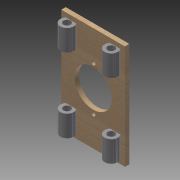
# Autodesk Inventor part: X_Carriage_WithBearings
Saved by Autodesk Inventor 2014 (Build 180170000, 170)
## iProperties
Created: 2013-12-16
Part Number: X_Carriage_WithBearings
Material: Ash
Document SubType Name: Modeling
Designer: Bram
Density: 0.641 g/cm^3
Appearance: Ash Door
Author: Bram
Autodesk Inventor part; units mm, degrees
ref_plane "YZ Plane" through (0, 0, 0) normal (1, 0, 0) x (0, 1, 0)
ref_plane "XZ Plane" through (0, 0, 0) normal (0, 1, 0) x (-1, 0, 0)
ref_plane "XY Plane" through (0, 0, 0) normal (0, 0, 1) x (1, 0, 0)
sketch "Sketch1" plane through (0, 0, 0) normal (0, 1, 0) x (-1, 0, 0)
  circle A0 centre (0, 0) radius 21
  circle A1 centre (0, 25) radius 2.5
  circle A2 centre (0, -25) radius 2.5
  line L0 (-31, 54) -> (-19, 54)
  line L1 (-19, 54) -> (-19, 30)
  line L2 (-19, 30) -> (-31, 30)
  line L3 (-31, 30) -> (-31, 54)
  line L4 (19, 54) -> (31, 54)
  line L5 (31, 54) -> (31, 30)
  line L6 (31, 30) -> (19, 30)
  line L7 (19, 30) -> (19, 54)
  line L8 (-31, -30) -> (-19, -30)
  line L9 (-19, -30) -> (-19, -54)
  line L10 (-19, -54) -> (-31, -54)
  line L11 (-31, -54) -> (-31, -30)
  line L12 (19, -30) -> (31, -30)
  line L13 (31, -30) -> (31, -54)
  line L14 (31, -54) -> (19, -54)
  line L15 (19, -54) -> (19, -30)
  line L16 (-36, 59) -> (36, 59)
  line L17 (36, 59) -> (36, -59)
  line L18 (36, -59) -> (-36, -59)
  line L19 (-36, -59) -> (-36, 59)
  dimension "d2" = 5
  dimension "d4" = 5
  dimension "d9" = 12
  dimension "d10" = 24
  dimension "d11" = 12
  dimension "d12" = 24
  dimension "d13" = 12
  dimension "d14" = 24
  dimension "d15" = 12
  dimension "d16" = 24
  constraints: 40 end point, 10 parallel, 5 horizontal, 5 perpendicular, 3 centre point
  measures "d2" diameter of A1
  measures "d4" diameter of A2
  measures "d9" distance of L1.end L2.end
  measures "d10" distance of L0.end L1.end
  measures "d11" distance of L6.start L6.end
  measures "d12" distance of L5.start L6.start
  measures "d13" distance of L10.start L10.end
  measures "d14" distance of L9.start L10.start
  measures "d15" distance of L14.start L14.end
  measures "d16" distance of L13.start L14.start
extrude "Extrusion1" add sketch "Sketch1" along normal blind 5
sketch "Sketch2" plane through (-31, 0, 30) normal (0, 0, 1) x (1, 0, 0)
  line L0 (12, 0) -> (0, 0) projected
  line L1 (0, 0) -> (0, 5) projected
  line L2 (6, 0) -> (6, -4.5)
  circle A0 centre (6, -4.5) radius 7.5
  circle A1 centre (6, -4.5) radius 4
  point P0 (31, 0)
  dimension "d23" = 4.5
  dimension "d24" = 15
  dimension "d25" = 8
  constraints: 2 centre point, 2 coincident, 2 end point, 1 midpoint, 1 parallel
  measures "d23" distance of L2.start L2.end
  measures "d24" diameter of A0
  measures "d25" diameter of A1
extrude "Extrusion2" add sketch "Sketch2" along normal blind 24
sketch "Sketch3" plane through (19, 0, 30) normal (0, 0, 1) x (1, 0, 0)
  line L0 (12, 0) -> (0, 0) projected
  line L1 (0, 0) -> (0, 5) projected
  line L2 (6, 0) -> (6, -4.5)
  circle A0 centre (6, -4.5) radius 7.5
  circle A1 centre (6, -4.5) radius 4
  point P0 (-19, 0)
  dimension "d28" = 4.5
  dimension "d29" = 15
  dimension "d30" = 8
  constraints: 2 centre point, 2 coincident, 2 end point, 1 midpoint, 1 parallel
  measures "d28" distance of L2.start L2.end
  measures "d29" diameter of A0
  measures "d30" diameter of A1
extrude "Extrusion3" add sketch "Sketch3" along normal blind 24
sketch "Sketch4" plane through (-19, 0, -30) normal (0, 0, -1) x (-1, 0, 0)
  line L0 (12, 0) -> (0, 0) projected
  line L1 (0, 0) -> (0, 5) projected
  line L2 (6, 0) -> (6, -4.5)
  circle A0 centre (6, -4.5) radius 4
  circle A1 centre (6, -4.5) radius 7.5
  point P0 (-19, 0)
  dimension "d33" = 4.5
  dimension "d34" = 8
  dimension "d35" = 15
  constraints: 2 centre point, 2 coincident, 2 end point, 1 midpoint, 1 parallel
  measures "d33" distance of L2.start L2.end
  measures "d34" diameter of A0
  measures "d35" diameter of A1
extrude "Extrusion4" add sketch "Sketch4" along normal blind 24
sketch "Sketch5" plane through (31, 0, -30) normal (0, 0, -1) x (-1, 0, 0)
  line L0 (12, 0) -> (0, 0) projected
  line L1 (0, 0) -> (0, 5) projected
  line L2 (6, 0) -> (6, -4.5)
  circle A0 centre (6, -4.5) radius 4
  circle A1 centre (6, -4.5) radius 7.5
  point P0 (31, 0)
  dimension "d38" = 4.5
  dimension "d39" = 8
  dimension "d40" = 15
  constraints: 2 centre point, 2 coincident, 2 end point, 1 midpoint, 1 parallel
  measures "d38" distance of L2.start L2.end
  measures "d39" diameter of A0
  measures "d40" diameter of A1
extrude "Extrusion5" add sketch "Sketch5" along normal blind 24
body "Solid1"
